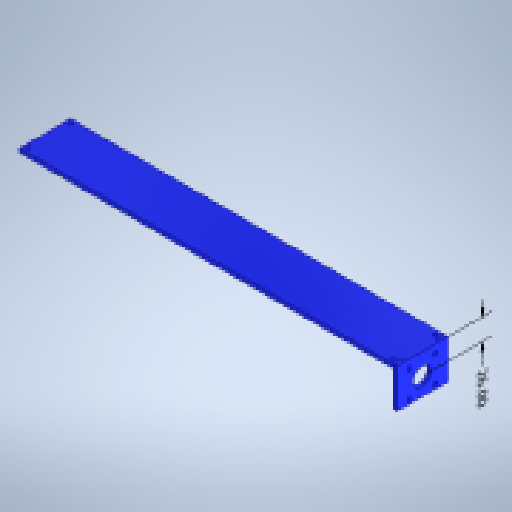
# Autodesk Inventor part: SoporteElectromecánico
Saved by Autodesk Inventor 2023 (Build 270158000, 158)
## iProperties
Created: 2023-04-07
Part Number: SoporteElectromecánico
Material: Steel, Mild, Welded
Document SubType Name: Modeling
Designer: Lenovo
Density: 7.85 g/cm^3
Appearance: Blue - Wall Paint - Glossy
Author: Lenovo
Autodesk Inventor part; units mm, degrees
ref_plane "YZ Plane" through (0, 0, 0) normal (1, 0, 0) x (0, 1, 0)
ref_plane "XZ Plane" through (0, 0, 0) normal (0, 1, 0) x (-1, 0, 0)
ref_plane "XY Plane" through (0, 0, 0) normal (0, 0, 1) x (1, 0, 0)
sketch "Sketch1" plane through (0, 0, 0) normal (1, 0, 0) x (0, 1, 0)
  arc A0 (8.8122, -5.4272) -> (7.5394, -4.9) centre (7.5394, -6.7) ccw
  line L0 (8.8122, -5.4272) -> (10.3168, -6.9318)
  arc A1 (9.9986, -7.7) -> (10.3168, -6.9318) centre (9.9986, -7.25) ccw
  line L1 (9.9986, -7.7) -> (8.8, -7.7)
  arc A2 (8.8, -7.7) -> (8.5, -8) centre (8.8, -8) ccw
  line L2 (8.5, -8) -> (8.5, -8.1257)
  arc A3 (8.5, -8.1257) -> (8.5879, -8.3379) centre (8.8, -8.1257) ccw
  line L3 (8.5879, -8.3379) -> (9.25, -9)
  line L4 (9.25, -9) -> (18, -9)
  line L5 (4.75, -9) -> (5.4121, -8.3379)
  arc A4 (5.4121, -8.3379) -> (5.5, -8.1257) centre (5.2, -8.1257) ccw
  line L6 (5.5, -8.1257) -> (5.5, -8)
  arc A5 (5.5, -8) -> (5.2, -7.7) centre (5.2, -8) ccw
  line L7 (5.2, -7.7) -> (4.0014, -7.7)
  arc A6 (3.6832, -6.9318) -> (4.0014, -7.7) centre (4.0014, -7.25) ccw
  line L8 (3.6832, -6.9318) -> (5.1878, -5.4272)
  arc A7 (6.4606, -4.9) -> (5.1878, -5.4272) centre (6.4606, -6.7) ccw
  line L9 (6.4606, -4.9) -> (7.5394, -4.9)
  line L10 (-4.75, -9) -> (4.75, -9)
  line L11 (-5.4121, -8.3379) -> (-4.75, -9)
  arc A8 (-5.5, -8.1257) -> (-5.4121, -8.3379) centre (-5.2, -8.1257) ccw
  arc A9 (-5.2, -7.7) -> (-5.5, -8) centre (-5.2, -8) ccw
  line L12 (-4.0014, -7.7) -> (-5.2, -7.7)
  arc A10 (-4.0014, -7.7) -> (-3.6832, -6.9318) centre (-4.0014, -7.25) ccw
  line L13 (-5.1878, -5.4272) -> (-3.6832, -6.9318)
  arc A11 (-5.1878, -5.4272) -> (-6.4606, -4.9) centre (-6.4606, -6.7) ccw
  line L14 (-7.5394, -4.9) -> (-6.4606, -4.9)
  arc A12 (-7.5394, -4.9) -> (-8.8122, -5.4272) centre (-7.5394, -6.7) ccw
  line L15 (-10.3168, -6.9318) -> (-8.8122, -5.4272)
  line L16 (-18, -9) -> (-9.25, -9)
  line L17 (-9.25, -9) -> (-8.5879, -8.3379)
  line L18 (-5.5, -8) -> (-5.5, -8.1257)
  line L19 (-8.5, -8.1257) -> (-8.5, -8)
  arc A13 (-8.5879, -8.3379) -> (-8.5, -8.1257) centre (-8.8, -8.1257) ccw
  arc A14 (-8.5, -8) -> (-8.8, -7.7) centre (-8.8, -8) ccw
  line L20 (-8.8, -7.7) -> (-9.9986, -7.7)
  arc A15 (-10.3168, -6.9318) -> (-9.9986, -7.7) centre (-9.9986, -7.25) ccw
  line L21 (18, -9) -> (21, -9)
  line L22 (21, -9) -> (21, -14)
  line L23 (-18, -9) -> (-21, -9)
  line L24 (-21, -9) -> (-21, -14)
  line L25 (-21, -14) -> (21, -14)
  line L26 (21, -14) -> (31, -14)
  line L27 (31, -14) -> (31, -9)
  line L28 (31, -9) -> (21, -9)
  line L29 (-21, -14) -> (-31, -14)
  line L30 (-31, -14) -> (-31, -9)
  line L31 (-31, -9) -> (-21, -9)
  line L32 (-21, -14) -> (-21, -9)
  line L33 (21, -14) -> (21, -9)
  point P0 (0, 0)
  dimension "d0" = 5
  dimension "d7" = 10
  dimension "d9" = 10
  constraints: 68 end point, 32 point on circle, 16 centre point, 7 perpendicular, 3 horizontal, 2 parallel, 1 point on line, 1 vertical
  measures "d0" distance of L21.end L25.end
  measures "d7" distance of L25.end L26.end
  measures "d9" distance of L25.start L29.end
extrude "Extrusion1" add sketch "Sketch1" along normal blind 456.6 contours L0 A1 L1 A2 L2 A3 L3 L4 L21 L22 L25 L24 L23 L16 L17 A13 L19 A14 L20 A15 L15 A12 L14 A11 L13 A10 L12 A9 L18 A8 L11 L10 L5 A4 L6 A5 L7 A6 L8 A7 L9 A0
sketch "Sketch2" plane through (0, 0, 0) normal (-1, 0, 0) x (0, 0, 1)
  circle A0 centre (-4.25, 15.7) radius 2.5
  circle A1 centre (28.25, 15.7) radius 2.5
  circle A2 centre (12, -0.55) radius 11
  circle A3 centre (28.25, -16.8) radius 2.5
  circle A4 centre (-4.25, -16.8) radius 2.5
  line L0 (-14, -21) -> (-14, 21) projected
  line L1 (-14, -21) -> (-9, -21)
  line L2 (-9, 21) -> (-14, 21)
  line L3 (-14, 21) -> (-14, -21)
  line L4 (33.45, 21) -> (33.45, -21)
  line L5 (33.45, -21) -> (-9.45, -21)
  line L6 (-9.45, 21) -> (33.45, 21)
  line L7 (-9, -9.25) -> (-9, -21) projected
  line L8 (33.45, -21) -> (-9, -21)
  line L9 (-13.9998, -20.9997) -> (-13.9998, -30.9997)
  line L10 (-9, -31) -> (33.45, -31)
  line L11 (33.45, -31) -> (33.45, -21)
  line L12 (33.45, 21) -> (-9, 21)
  line L13 (-14, 21) -> (-9, 21) projected
  line L14 (-13.9998, 21.0003) -> (-13.9998, 31.0003)
  line L15 (-9, 31) -> (33.45, 31)
  line L16 (33.45, 31) -> (33.45, 21)
  line L17 (-13.9998, -30.9997) -> (33.45, -30.9997)
  line L18 (33.45, -30.9997) -> (33.45, -21)
  line L19 (33.45, -21) -> (-13.9998, -21)
  line L20 (-13.9998, -21) -> (-13.9998, -30.9997)
  line L21 (33.45, 21) -> (-13.9998, 21)
  line L22 (-13.9998, 21) -> (-13.9998, 31.0003)
  line L23 (-13.9998, 31.0003) -> (33.45, 31.0003)
  line L24 (33.45, 31.0003) -> (33.45, 21)
  point P0 (12, -11.55)
  point P1 (-14, 21)
  point P2 (-13.9998, -21)
  dimension "d12" = 11.18
  dimension "d13" = 11.1805
  constraints: 44 end point, 9 perpendicular, 6 parallel, 5 centre point, 4 horizontal, 2 point on line
  measures "d12" distance of L1.end L9.end
  measures "d13" distance of L2.start L14.end
extrude "Extrusion2" add sketch "Sketch2" along normal blind 5 contours L0 L2 L6 L4 L5 L1
extrude "Extrusion3" add sketch "Sketch1" along normal up to surface (456.6 mm away) contours L28 L27 L26 L22 | L29 L30 L31 L24
extrude "Extrusion4" add sketch "Sketch2" along normal up to surface (5 mm away) contours L1 L5 L11 L10 L17 L9 | L14 L23 L15 L16 L6 L2
sketch "Sketch3" plane through (-5, -21, -14) normal (0, 0, -1) x (-1, 0, 0)
  line L0 (-461.6, -10) -> (-461.6, 0) projected
  line L1 (-461.6, -10) -> (-451.6, -10)
  line L2 (-451.6, -10) -> (-451.6, 0)
  line L3 (-451.6, 0) -> (-461.6, 0)
  line L4 (-461.6, 0) -> (-461.6, -10)
  line L5 (-5, -10) -> (-461.6, -10) projected
  line L6 (-461.6, -10) -> (-451.6, 0)
  line L7 (-5, 0) -> (-461.6, 0) projected
  line L8 (-461.6, 0) -> (-451.6, -10)
  circle A0 centre (-456.6, -5) radius 2.5
  line L9 (-5, 52) -> (-461.6, 52) projected
  line L10 (-461.6, 52) -> (-451.6, 52)
  line L11 (-451.6, 52) -> (-451.6, 42)
  line L12 (-451.6, 42) -> (-461.6, 42)
  line L13 (-461.6, 42) -> (-461.6, 52)
  line L14 (-461.6, 42) -> (-451.6, 52)
  line L15 (-461.6, 52) -> (-451.6, 42)
  circle A1 centre (-456.6, 47) radius 2.5
  line L16 (0, -9.9997) -> (0, 0) projected
  line L17 (0, -9.9997) -> (-20, -9.9997)
  line L18 (-20, -9.9997) -> (-20, 0.0003)
  line L19 (-20, 0.0003) -> (0, 0.0003)
  line L20 (0, 0.0003) -> (0, -9.9997)
  line L21 (-5, 0) -> (0, 0) projected
  line L22 (-20, -9.9997) -> (0, 0)
  line L23 (0, 0) -> (-20, 0.0003)
  line L24 (-20, 0.0003) -> (0, -9.9997)
  circle A2 centre (-10, -4.9997) radius 2.5
  line L25 (0, 52.0003) -> (0, -9.9997) projected
  line L26 (0, 52.0003) -> (-20, 52.0003)
  line L27 (-20, 52.0003) -> (-20, 42.0003)
  line L28 (-20, 42.0003) -> (0, 42.0003)
  line L29 (0, 42.0003) -> (0, 52.0003)
  line L30 (-20, 42.0003) -> (0, 52.0003)
  line L31 (-20, 52.0003) -> (0, 42.0003)
  circle A3 centre (-10, 47.0003) radius 2.5
  point P0 (-5, 21)
  dimension "d22" = 10
  dimension "d23" = 10
  dimension "d24" = 5
  dimension "d25" = 10
  dimension "d26" = 10
  dimension "d27" = 5
  dimension "d28" = 20
  dimension "d29" = 10
  dimension "d30" = 5
  dimension "d31" = 20
  dimension "d32" = 10
  dimension "d33" = 5
  constraints: 50 end point, 8 parallel, 5 midpoint, 5 perpendicular, 4 centre point, 4 horizontal, 1 point on line
  measures "d22" distance of L3.end L2.end
  measures "d23" distance of L2.end L1.end
  measures "d24" diameter of A0
  measures "d25" distance of L11.end L12.end
  measures "d26" distance of L10.end L11.end
  measures "d27" diameter of A1
  measures "d28" distance of L18.end L19.end
  measures "d29" distance of L17.end L18.end
  measures "d30" diameter of A2
  measures "d31" distance of L28.end L27.end
  measures "d32" distance of L27.end L26.end
  measures "d33" diameter of A3
extrude "Extrusion5" cut sketch "Sketch3" against normal through all contours A0 L8 L6 | L6 L8 A0 | A0 L6 L8 | L8 L6 A0 | A2 L24 L22 | L22 L24 A2 | A2 L22 L24 | L22 A2 L24 | A3 L30 L31 | L31 L30 A3 | L30 L31 A3 | A3 L31 L30 | A1 L15 L14 | L14 L15 A1 | L15 L14 A1 | A1 L14 L15
body "Solid1"
